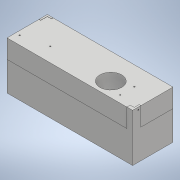
# Autodesk Inventor part: 5руб
Saved by Autodesk Inventor 2020 (Build 240168000, 168)
## iProperties
Created: 2020-02-01
Part Number: 5руб
Material: Типовые
Document SubType Name: Modeling
Designer: Css38
Density: 1 g/cm^3
Appearance: По умолчанию
Author: Css38
Autodesk Inventor part; units mm, degrees
ref_plane "YZ Plane" through (0, 0, 0) normal (1, 0, 0) x (0, 1, 0)
ref_plane "XZ Plane" through (0, 0, 0) normal (0, 1, 0) x (-1, 0, 0)
sketch "Эскиз1" plane through (0, 0, 0) normal (0, 0, 1) x (1, 0, 0)
  line L0 (-76.25, 24.5) -> (76.25, 24.5)
  line L1 (76.25, 24.5) -> (76.25, -24.5)
  line L2 (76.25, -24.5) -> (-76.25, -24.5)
  line L3 (-76.25, -24.5) -> (-76.25, 24.5)
  line L4 (-76.25, 24.5) -> (76.25, -24.5) construction
  line L5 (76.25, 24.5) -> (-76.25, -24.5) construction
  point P0 (0, 0)
  point P1 (0, 0)
  dimension "d35" = 152.5
  dimension "d36" = 49
  constraints: 12 end point, 2 parallel, 1 coincident, 1 horizontal, 1 midpoint, 1 perpendicular
  measures "d35" distance of L1.end L2.end
  measures "d36" distance of L2.end L0.start
extrude "Выдавливание1" add sketch "Эскиз1" along normal blind 30
sketch "Эскиз2" plane through (0, 0, 30) normal (0, 0, 1) x (1, 0, 0)
  line L0 (76.25, 24.5) -> (76.25, -24.5) construction
  line L1 (76.25, -24.5) -> (-76.25, -24.5) construction
  line L2 (-76.25, -24.5) -> (-76.25, 24.5) construction
  line L3 (-76.25, 24.5) -> (76.25, 24.5) construction
  line L4 (74.25, -20.5) -> (47.25, -20.5)
  line L5 (47.25, -20.5) -> (47.25, 6.5)
  line L6 (47.25, 6.5) -> (74.25, 6.5)
  line L7 (74.25, 6.5) -> (74.25, -20.5)
  point P0 (0, 0)
  dimension "d40" = 27
  dimension "d137" = 2
  dimension "d138" = 4
  constraints: 8 end point, 2 parallel, 2 perpendicular, 1 horizontal
  measures "d40" distance of L5.end L6.end
  measures "d137" distance between parallel lines of L0 L7
  measures "d138" distance between parallel lines of L4 L1
extrude "Выдавливание2" cut sketch "Эскиз2" against normal up to next
sketch "Эскиз3" plane through (0, 0, 30) normal (0, 0, 1) x (1, 0, 0)
  line L0 (47.25, 6.5) -> (47.25, -20.5)
  line L1 (47.25, -20.5) -> (74.25, -20.5)
  line L2 (74.25, -20.5) -> (74.25, 6.5)
  line L3 (74.25, 6.5) -> (47.25, 6.5)
  line L4 (76.25, 24.5) -> (76.25, -24.5) construction
  line L5 (76.25, -24.5) -> (-76.25, -24.5) construction
  line L6 (-76.25, 24.5) -> (76.25, 24.5) construction
  line L7 (76.25, 24.5) -> (-76.25, 24.5) projected
  line L8 (-76.25, 24.5) -> (76.25, 24.5)
  line L9 (76.25, 24.5) -> (76.25, -24.5)
  line L10 (76.25, -24.5) -> (-76.25, -24.5)
  line L11 (-76.25, 24.5) -> (-76.25, 22.5)
  line L12 (-76.25, 24.5) -> (-76.25, -24.5) construction
  line L13 (-76.25, 22.5) -> (-2.75, 22.5)
  line L14 (-2.75, 22.5) -> (-2.75, 6.5)
  line L15 (-2.75, 6.5) -> (17.25, 6.5)
  line L16 (17.25, 6.5) -> (17.25, -20.5)
  line L17 (17.25, -20.5) -> (-76.25, -20.5)
  line L18 (-76.25, -24.5) -> (-76.25, -20.5)
  line L19 (-76.25, -24.5) -> (76.25, -24.5) projected
  line L20 (76.25, -24.5) -> (76.25, 24.5) projected
  line L21 (74.25, -20.5) -> (47.25, -20.5) projected
  line L22 (47.25, -20.5) -> (47.25, 6.5) projected
  line L23 (47.25, 6.5) -> (74.25, 6.5) projected
  line L24 (74.25, 6.5) -> (74.25, -20.5) projected
  dimension "d50" = 2
  dimension "d52" = 20
  dimension "d63" = 30
  constraints: 34 end point, 13 collinear, 4 perpendicular, 2 parallel, 2 point on line
  measures "d50" distance of L6.start L11.end
  measures "d52" distance between parallel lines of L14 L16
  measures "d63" distance between parallel lines of L0 L16
extrude "Выдавливание4" add sketch "Эскиз3" along normal blind 3
sketch "Эскиз4" plane through (0, 0, 33) normal (0, 0, 1) x (1, 0, 0)
  line L0 (47.25, 6.5) -> (47.25, -20.5) construction
  line L1 (47.25, -20.5) -> (74.25, -20.5) construction
  line L2 (74.25, -20.5) -> (74.25, 6.5) construction
  line L3 (74.25, 6.5) -> (47.25, 6.5) construction
  line L4 (76.25, 24.5) -> (76.25, -24.5) projected
  line L5 (76.25, -24.5) -> (-76.25, -24.5) projected
  line L6 (-76.25, -24.5) -> (-76.25, -20.5) projected
  line L7 (-76.25, -20.5) -> (17.25, -20.5) projected
  line L8 (17.25, -20.5) -> (17.25, 6.5) projected
  line L9 (17.25, 6.5) -> (-2.75, 6.5) projected
  line L10 (-2.75, 6.5) -> (-2.75, 22.5) projected
  line L11 (-2.75, 22.5) -> (-76.25, 22.5) projected
  line L12 (-76.25, 22.5) -> (-76.25, 24.5) projected
  line L13 (-76.25, 24.5) -> (76.25, 24.5) projected
  line L14 (17.25, -20.5) -> (17.25, 6.5) projected
  line L15 (17.25, 6.5) -> (47.25, 6.5) construction
  line L16 (47.25, 6.5) -> (47.25, -20.5) projected
  line L17 (47.25, -20.5) -> (17.25, -20.5) construction
  circle A0 centre (32.25, -7) radius 13.25
  line L18 (32.25, -7) -> (32.25, 6.5) construction
  line L19 (32.25, -7) -> (32.25, -20.5) construction
  line L20 (47.25, -20.5) -> (47.25, 6.5) construction
  line L21 (32.25, -7) -> (17.25, -7) construction
  line L22 (32.25, -7) -> (47.25, -7) construction
  point P0 (0, 0)
  dimension "d55" = 26.5
  constraints: 12 end point, 4 midpoint, 3 perpendicular, 2 collinear, 1 centre point, 1 point on line, 1 other
  measures "d55" diameter of A0
extrude "Выдавливание7" add sketch "Эскиз4" along normal blind 25
sketch "Эскиз6" plane through (17.25, -20.5, 30) normal (-1, 0, 0) x (0, 0, 1)
  line L0 (3, 0.25) -> (3, 26.75) construction
  line L1 (0, 27) -> (28, 27) projected
  line L2 (0, 0) -> (28, 0) projected
  line L3 (3, 27) -> (5.4, 27)
  line L4 (5.4, 27) -> (5.4, 0)
  line L5 (5.4, 0) -> (3, 0)
  line L6 (3, 0) -> (3, 27)
  point P0 (-30, 20.5)
  dimension "d66" = 2.4
  constraints: 8 end point, 2 parallel, 2 point on line, 1 collinear, 1 horizontal, 1 perpendicular
  measures "d66" distance of L4.end L5.end
extrude "Выдавливание8" cut sketch "Эскиз6" against normal up to surface (57 mm away) from surface at 0
sketch "Эскиз7" plane through (0, 0, 58) normal (0, 0, 1) x (1, 0, 0)
  line L0 (76.25, -24.5) -> (-76.25, -24.5) projected
  line L1 (-76.25, 24.5) -> (76.25, 24.5) projected
  line L2 (76.25, -24.5) -> (-76.25, -24.5)
  line L3 (-76.25, -24.5) -> (-76.25, 24.5)
  line L4 (-76.25, 24.5) -> (76.25, 24.5)
  line L5 (76.25, 24.5) -> (76.25, -24.5)
  circle A0 centre (32.25, -7) radius 13.25 projected
  point P0 (0, 0)
  constraints: 8 end point, 2 parallel, 1 horizontal, 1 perpendicular
extrude "Выдавливание9" add sketch "Эскиз7" against normal blind 17.15
ref_plane "РабПлоскость1" through (74.25, -20.5, 35.4) normal (0, 0, -1) x (-1, 0, 0)
split body "Разделение1" result two bodies by plane through (74.25, -20.5, 35.4) normal (0, 0, -1) first body at (-35.0833, 2.1667, 0.5)
sketch "Эскиз21" plane through (0, 0, 30) normal (0, 0, 1) x (1, 0, 0)
  line L0 (-76.25, -20.5) -> (17.25, -20.5) construction
  line L1 (17.25, -20.5) -> (17.25, 6.5) construction
  line L2 (17.25, 6.5) -> (-2.75, 6.5) construction
  line L3 (-2.75, 6.5) -> (-2.75, 22.5) construction
  line L4 (-2.75, 22.5) -> (-76.25, 22.5) construction
  line L5 (-76.25, -20.5) -> (-76.25, 22.5) construction
  line L6 (-76.25, -24.5) -> (-76.25, -20.5) construction
  line L7 (76.25, -24.5) -> (-76.25, -24.5) construction
  line L8 (76.25, 24.5) -> (76.25, -24.5) construction
  line L9 (74.25, 6.5) -> (47.25, 6.5) construction
  line L10 (47.25, 6.5) -> (47.25, -20.5) construction
  line L11 (47.25, -20.5) -> (74.25, -20.5) construction
  line L12 (74.25, -20.5) -> (74.25, 6.5) construction
  line L13 (-76.25, -20.5) -> (-43.25, -20.5)
  line L14 (-43.25, -20.5) -> (-43.25, -8)
  line L15 (-43.25, -8) -> (-76.25, -8)
  line L16 (-76.25, -8) -> (-76.25, -20.5)
  line L17 (-76.25, 22.5) -> (-76.25, 24.5) projected
  line L18 (-76.25, 24.5) -> (76.25, 24.5) projected
  point P0 (0, 0)
  dimension "d139" = 33
  dimension "d140" = 12.5
  constraints: 8 end point, 2 parallel, 1 horizontal, 1 perpendicular
  measures "d139" distance of L15.end L14.end
  measures "d140" distance of L14.end L13.end
extrude "Выдавливание26" cut sketch "Эскиз21" against normal blind 28 bodies 2
sketch "Эскиз22" plane through (0, 0, 2) normal (0, 0, 1) x (1, 0, 0)
  line L0 (76.25, 24.5) -> (76.25, -24.5) construction
  line L1 (76.25, -24.5) -> (-76.25, -24.5) construction
  line L2 (-76.25, -24.5) -> (-76.25, -20.5) construction
  line L3 (-76.25, -20.5) -> (-76.25, -8) construction
  line L4 (-43.25, -8) -> (-76.25, -8) construction
  line L5 (-43.25, -20.5) -> (-43.25, -8) construction
  line L6 (-76.25, -20.5) -> (-43.25, -20.5) construction
  line L7 (-76.25, -8) -> (-76.25, 24.5) construction
  line L8 (74.25, 6.5) -> (47.25, 6.5) construction
  line L9 (47.25, 6.5) -> (47.25, -20.5) construction
  line L10 (47.25, -20.5) -> (74.25, -20.5) construction
  line L11 (74.25, -20.5) -> (74.25, 6.5) construction
  line L12 (-43.25, -8) -> (-47.75, -8)
  line L13 (-47.75, -8) -> (-47.75, -20.5)
  line L14 (-47.75, -20.5) -> (-43.25, -20.5)
  line L15 (-43.25, -20.5) -> (-43.25, -8)
  line L16 (-76.25, 24.5) -> (76.25, 24.5) projected
  point P0 (0, 0)
  dimension "d143" = 4.5
  constraints: 8 end point, 2 parallel, 1 horizontal, 1 perpendicular, 1 point on line
  measures "d143" distance of L14.end L13.end
extrude "Выдавливание27" add sketch "Эскиз22" along normal blind 18 bodies 2
sketch "Эскиз23" plane through (0, 0, 20) normal (0, 0, 1) x (1, 0, 0)
  line L0 (76.25, 24.5) -> (76.25, -24.5) construction
  line L1 (76.25, -24.5) -> (-76.25, -24.5) construction
  line L2 (-76.25, -24.5) -> (-76.25, -20.5) construction
  line L3 (-76.25, -20.5) -> (-47.75, -20.5) construction
  line L4 (-47.75, -20.5) -> (-47.75, -8) construction
  line L5 (-43.25, -8) -> (-47.75, -8) construction
  line L6 (-43.25, -20.5) -> (-43.25, -8) construction
  line L7 (-47.75, -20.5) -> (-43.25, -20.5) construction
  line L8 (-76.25, -8) -> (-76.25, 24.5) construction
  line L9 (-47.75, -8) -> (-76.25, -8) construction
  line L10 (74.25, 6.5) -> (47.25, 6.5) construction
  line L11 (47.25, 6.5) -> (47.25, -20.5) construction
  line L12 (47.25, -20.5) -> (74.25, -20.5) construction
  line L13 (74.25, -20.5) -> (74.25, 6.5) construction
  line L14 (-43.25, -20.5) -> (-47.75, -8) construction
  line L15 (-43.25, -8) -> (-47.75, -20.5) construction
  circle A0 centre (-45.5, -14.25) radius 0.75
  line L16 (-76.25, 24.5) -> (76.25, 24.5) projected
  point P0 (0, 0)
  dimension "d146" = 1.5
  constraints: 4 end point, 1 centre point, 1 midpoint
  measures "d146" diameter of A0
extrude "Выдавливание28" cut sketch "Эскиз23" against normal blind 3 bodies 2
sketch "Эскиз24" plane through (0, 0, 30) normal (0, 0, 1) x (1, 0, 0)
  line L0 (76.25, 24.5) -> (76.25, -24.5) construction
  line L1 (76.25, -24.5) -> (-76.25, -24.5) construction
  line L2 (-76.25, -24.5) -> (-76.25, -20.5) construction
  line L3 (-76.25, -20.5) -> (-43.25, -20.5) construction
  line L4 (-43.25, -20.5) -> (-43.25, -8) construction
  line L5 (-43.25, -8) -> (-76.25, -8) construction
  line L6 (-76.25, -8) -> (-76.25, 22.5) construction
  line L7 (-43.25, -20.5) -> (17.25, -20.5) construction
  line L8 (17.25, -20.5) -> (17.25, 6.5) construction
  line L9 (17.25, 6.5) -> (-2.75, 6.5) construction
  line L10 (-2.75, 6.5) -> (-2.75, 22.5) construction
  line L11 (-2.75, 22.5) -> (-76.25, 22.5) construction
  line L12 (74.25, 6.5) -> (47.25, 6.5) construction
  line L13 (47.25, 6.5) -> (47.25, -20.5) construction
  line L14 (47.25, -20.5) -> (74.25, -20.5) construction
  line L15 (74.25, -20.5) -> (74.25, 6.5) construction
  line L16 (-43.25, -8) -> (-43.25, -20.5) construction
  line L17 (-65.25, -14.25) -> (-49.3603, 16.9352)
  line L18 (-49.3603, 16.9352) -> (-31.2743, -7)
  line L19 (-31.2743, -7) -> (17.7257, -7)
  line L20 (-76.25, 22.5) -> (-76.25, 24.5) projected
  line L21 (-76.25, 24.5) -> (76.25, 24.5) projected
  point P0 (0, 0)
  point P1 (-43.25, -14.25)
  point P2 (47.25, -7)
  dimension "d149" = 11
  dimension "d150" = 35
  dimension "d151" = 49
  dimension "d152" = 63
  dimension "d153" = 30
  constraints: 6 end point, 2 midpoint, 1 horizontal, 1 horizontal alignment, 1 point on line
  measures "d149" distance from line of L2 L17.start
  measures "d150" distance of L17.start L17.end
  measures "d151" distance of L18.end L19.end
  measures "d152" angle of L7 L17
  measures "d153" distance of L17.end L18.end
sketch "Эскиз20" plane through (0, 0, 58) normal (0, 0, 1) x (1, 0, 0)
  line L0 (-46, -24.5) -> (57.5, -24.5) construction
  line L1 (57.5, -24.5) -> (57.5, 10) construction
  line L2 (57.5, 10) -> (47.5, 10) construction
  line L3 (-46, 10) -> (-46, -24.5) construction
  circle A0 centre (32.25, -7) radius 13.25 construction
  line L4 (47.5, 10) -> (47.5, -24.5) construction
  line L5 (-76.25, -24.5) -> (76.25, -24.5) construction
  line L6 (-76.25, -24.5) -> (76.25, -24.5) construction
  line L7 (-76.25, 24.5) -> (-76.25, -24.5) construction
  circle A1 centre (-71.25, -14.2) radius 0.5
  line L8 (-36, 10) -> (-36, -24.5) construction
  line L9 (-36, 10) -> (-46, 10) construction
  line L10 (47.5, 10) -> (-36, 10) construction
  line L11 (-46, 10) -> (-36, -24.5) construction
  line L12 (-36, 10) -> (-46, -24.5) construction
  line L13 (57.5, 10) -> (47.5, -7.25) construction
  line L14 (47.5, -7.25) -> (57.5, -24.5) construction
  line L15 (47.5, -24.5) -> (57.5, -7.25) construction
  line L16 (57.5, -7.25) -> (47.5, 10) construction
  circle A2 centre (-41, -7.25) radius 0.5
  circle A3 centre (52.5, 1.375) radius 0.5
  circle A4 centre (52.5, -15.875) radius 0.5
  point P0 (0, 0)
  dimension "d129" = 34.5
  dimension "d131" = 10
  dimension "d154" = 5
  dimension "d155" = 10.3
  dimension "d156" = 2
  dimension "d157" = 103.5
  dimension "d158" = 1
  constraints: 28 end point, 5 midpoint, 5 parallel, 4 centre point, 3 equal radius, 2 collinear, 2 perpendicular, 2 point on line, 1 horizontal
  measures "d129" distance of L1.end L0.end
  measures "d131" distance between parallel lines of L1 L4
  measures "d154" distance from line of L7 A1.centre
  measures "d155" distance from line of L5 A1.centre
  measures "d156" distance edge to line of A0 L4
  measures "d157" distance of L1.end L3.start
  measures "d158" diameter of A2
hole "Отверстие1" at (-71.25, -14.2, 58) at (-41, -7.25, 58) at (52.5, 1.375, 58) at (52.5, -15.875, 58) direction (0, 0, -1) diameter 1 depth 4 tip angle 118 countersink diameter 1.5 countersink angle 90 bodies 3
sketch "Эскиз25" plane through (0, 0, 30) normal (0, 0, 1) x (1, 0, 0)
  line L0 (-76.25, -24.5) -> (-76.25, -20.5) construction
  line L1 (-76.25, -20.5) -> (-43.25, -20.5) construction
  line L2 (-43.25, -20.5) -> (-43.25, -8) construction
  line L3 (-43.25, -8) -> (-76.25, -8) construction
  line L4 (-76.25, -8) -> (-76.25, 22.5) construction
  line L5 (-76.25, 22.5) -> (-76.25, 24.5) construction
  line L6 (-76.25, 24.5) -> (76.25, 24.5) construction
  line L7 (76.25, 24.5) -> (76.25, -24.5) construction
  line L8 (76.25, -24.5) -> (-76.25, -24.5) construction
  line L9 (-43.25, -20.5) -> (17.25, -20.5) construction
  line L10 (17.25, -20.5) -> (17.25, 6.5) construction
  line L11 (17.25, 6.5) -> (-2.75, 6.5) construction
  line L12 (-2.75, 6.5) -> (-2.75, 22.5) construction
  line L13 (-2.75, 22.5) -> (-76.25, 22.5) construction
  line L14 (74.25, 6.5) -> (47.25, 6.5) construction
  line L15 (47.25, 6.5) -> (47.25, -20.5) construction
  line L16 (47.25, -20.5) -> (74.25, -20.5) construction
  line L17 (74.25, -20.5) -> (74.25, 6.5) construction
  line L18 (-76.25, 24.5) -> (-69.25, 24.5)
  line L19 (-69.25, 24.5) -> (-69.25, 22.5)
  line L20 (-69.25, 22.5) -> (-74.25, 22.5)
  line L21 (-74.25, 22.5) -> (-74.25, 14.5)
  line L22 (-74.25, 14.5) -> (-76.25, 14.5)
  line L23 (-76.25, 14.5) -> (-76.25, 24.5)
  line L24 (76.25, -24.5) -> (69.25, -24.5)
  line L25 (69.25, -24.5) -> (69.25, -20.5)
  line L26 (69.25, -20.5) -> (74.25, -20.5)
  line L27 (74.25, -20.5) -> (74.25, -14.5)
  line L28 (74.25, -14.5) -> (76.25, -14.5)
  line L29 (76.25, -14.5) -> (76.25, -24.5)
  point P0 (0, 0)
  dimension "d166" = 10
  dimension "d168" = 5
  constraints: 25 end point, 10 perpendicular, 3 parallel, 2 horizontal, 1 point on line
  measures "d166" distance of L5.end L22.end
  measures "d168" distance of L19.end L20.end
extrude "Выдавливание29" add sketch "Эскиз25" along normal blind 28.1 bodies 2
sketch "Эскиз26" plane through (76.25, -24.5, 0) normal (1, 0, 0) x (0, 0, -1)
  line L0 (0, 4) -> (-58.1, 4) construction
  line L1 (-58.1, 4) -> (-52.1, 10) construction
  line L2 (-35.4, 10) -> (-58.1, 10) construction
  line L3 (-58.1, 10) -> (-52.1, 4) construction
  circle A0 centre (-55.1, 7) radius 0.5
  point P0 (0, 24.5)
  dimension "d171" = 1
  constraints: 4 end point, 2 perpendicular, 2 point on line, 1 centre point, 1 midpoint
  measures "d171" diameter of A0
hole "Отверстие2" at (76.25, -17.5, 55.1) direction (-1, 0, 0) diameter 1 end through all countersink diameter 1.5 countersink angle 90 bodies 2
sketch "Эскиз27" plane through (-76.25, -24.5, 0) normal (-1, 0, 0) x (0, 0, 1)
  line L0 (58.1, 47) -> (30, 47) construction
  circle A0 centre (55.1, 7) radius 0.5 construction
  line L1 (35.4, 47) -> (58.1, 47) construction
  line L2 (58.1, 47) -> (50.1, 39) construction
  line L3 (30, 39) -> (58.1, 39) construction
  line L4 (58.1, 39) -> (50.1, 47) construction
  circle A1 centre (54.1, 43) radius 0.5
  point P0 (0, 24.5)
  constraints: 4 end point, 2 perpendicular, 2 point on line, 1 centre point, 1 equal radius, 1 midpoint
hole "Отверстие3" at (-76.25, 18.5, 54.1) direction (1, 0, 0) diameter 1 end through all countersink diameter 1.5 countersink angle 90 bodies 2
sketch "Эскиз28" plane through (0, 0, 58) normal (0, 0, 1) x (1, 0, 0)
  line L0 (69.25, -24.5) -> (69.25, -20.5) construction
  line L1 (69.25, -20.5) -> (74.25, -20.5) construction
  line L2 (74.25, -20.5) -> (74.25, -14.5) construction
  line L3 (74.25, -14.5) -> (76.25, -14.5) construction
  line L4 (76.25, -14.5) -> (76.25, -24.5) construction
  line L5 (76.25, -24.5) -> (69.25, -24.5) construction
  line L6 (-74.25, 22.5) -> (-74.25, 14.5) construction
  line L7 (-74.25, 14.5) -> (-76.25, 14.5) construction
  line L8 (-76.25, 14.5) -> (-76.25, 24.5) construction
  line L9 (-76.25, 24.5) -> (-69.25, 24.5) construction
  line L10 (-69.25, 24.5) -> (-69.25, 22.5) construction
  line L11 (-69.25, 22.5) -> (-74.25, 22.5) construction
  circle A0 centre (52.5, 1.375) radius 0.75 construction
  circle A1 centre (-71.25, -14.2) radius 0.75 construction
  circle A2 centre (-41, -7.25) radius 0.75 construction
  circle A3 centre (52.5, -15.875) radius 0.75 construction
  line L12 (-76.25, -24.5) -> (-76.25, 24.5) construction
  line L13 (-76.25, 24.5) -> (76.25, 24.5) construction
  line L14 (76.25, 24.5) -> (76.25, -24.5) construction
  line L15 (76.25, -24.5) -> (-76.25, -24.5) construction
  circle A4 centre (32.25, -7) radius 13.25 construction
  line L16 (-74.15, 22.4) -> (-74.15, 14.4)
  line L17 (-74.15, 14.4) -> (-76.35, 14.4)
  line L18 (-76.35, 14.4) -> (-76.35, 24.6)
  line L19 (-76.35, 24.6) -> (-69.15, 24.6)
  line L20 (-69.15, 24.6) -> (-69.15, 22.4)
  line L21 (-69.15, 22.4) -> (-74.15, 22.4)
  line L22 (74.15, -20.4) -> (69.15, -20.4)
  line L23 (69.15, -20.4) -> (69.15, -24.6)
  line L24 (69.15, -24.6) -> (76.35, -24.6)
  line L25 (76.35, -24.6) -> (76.35, -14.4)
  line L26 (76.35, -14.4) -> (74.15, -14.4)
  line L27 (74.15, -14.4) -> (74.15, -20.4)
  point P0 (0, 0)
  dimension "d186" = 0.1
  dimension "d187" = 0.1
  constraints: 24 end point, 10 other
  measures "d186" distance between parallel lines of L11 L21
  measures "d187" distance between parallel lines of L1 L22
extrude "Выдавливание30" cut sketch "Эскиз28" against normal through all bodies 3
sketch "Эскиз29" plane through (74.15, -20.4, 58) normal (1, 0, 0) x (0, 0, -1)
  circle A0 centre (2.9, 2.9) radius 0.5 construction
  circle A1 centre (3, 2.9) radius 0.5
  point P0 (58, 20.4)
  dimension "d190" = 0.1
  constraints: 1 centre point, 1 equal radius, 1 horizontal alignment
  measures "d190" distance of A0.centre A1.centre
hole "Отверстие4" at (74.15, -17.5, 55) direction (-1, 0, 0) diameter 1 depth 3 tip angle 118 countersink diameter 1.5 countersink angle 90 bodies 3
sketch "Эскиз30" plane through (-74.15, 14.4, 58) normal (-1, 0, 0) x (0, 0, 1)
  circle A0 centre (-3, -31.9) radius 0.5 construction
  circle A1 centre (-3, 4) radius 0.5
  line L0 (0, 8) -> (0, 0) construction
  point P0 (-58, -14.4)
  point P1 (0, 4)
  constraints: 1 centre point, 1 equal radius, 1 horizontal alignment, 1 midpoint, 1 vertical alignment
hole "Отверстие5" at (-74.15, 18.4, 55) direction (1, 0, 0) diameter 1 depth 3 tip angle 118 countersink diameter 1.5 countersink angle 90 bodies 3
